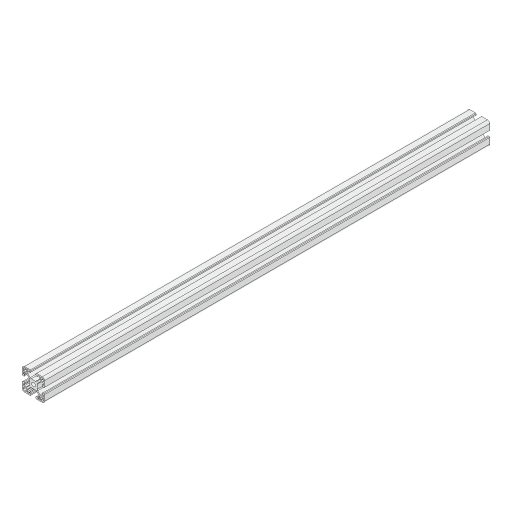
# Autodesk Inventor part: Al-profile-30x30
Saved by Autodesk Inventor 2023.1 (Build 271208000, 208)
## iProperties
Created: 2023-06-30
Part Number: Al-profile-30x30
Material: Aluminum 6061
Document SubType Name: Modeling
Designer: kuzmin
Density: 2.7 g/cm^3
Appearance: Aluminum - Flat
length: 600.000 mm
Author: kuzmin
Autodesk Inventor part; units mm, degrees
ref_plane "YZ Plane" through (0, 0, 0) normal (1, 0, 0) x (0, 1, 0)
ref_plane "XZ Plane" through (0, 0, 0) normal (0, 1, 0) x (-1, 0, 0)
ref_plane "XY Plane" through (0, 0, 0) normal (0, 0, 1) x (1, 0, 0)
sketch "Sketch1" plane through (0, 0, 0) normal (0, 0, 1) x (1, 0, 0)
  line L0 (5.2, -2.9574) -> (5.2, 2.9574) construction
  arc A0 (5.7858, 4.3716) -> (5.2, 2.9574) centre (7.2, 2.9574) ccw
  line L1 (5.7858, 4.3716) -> (9.0284, 7.6142)
  arc A1 (10.4426, 8.2) -> (9.0284, 7.6142) centre (10.4426, 6.2) ccw
  line L2 (10.4426, 8.2) -> (12.8, 8.2)
  arc A2 (13.6, 7.4) -> (12.8, 8.2) centre (12.8, 7.4) ccw
  line L3 (13.6, 7.4) -> (13.6, 6.1)
  arc A3 (13.3, 5.8) -> (13.6, 6.1) centre (13.3, 6.1) ccw
  line L4 (13.3, 5.8) -> (12.25, 5.8)
  arc A4 (12.25, 5.8) -> (11.95, 5.5) centre (12.25, 5.5) ccw
  line L5 (11.95, 5.5) -> (11.95, 4.2)
  arc A5 (11.95, 4.2) -> (12.75, 3.4) centre (12.75, 4.2) ccw
  line L6 (12.75, 3.4) -> (14.2, 3.4)
  arc A6 (14.2, 3.4) -> (15, 4.2) centre (14.2, 4.2) ccw
  line L7 (15, 4.2) -> (15, 12)
  arc A7 (15, 12) -> (12, 15) centre (12, 12) ccw
  line L8 (12, 15) -> (4.2, 15)
  arc A8 (4.2, 15) -> (3.4, 14.2) centre (4.2, 14.2) ccw
  line L9 (3.4, 14.2) -> (3.4, 12.75)
  arc A9 (3.4, 12.75) -> (4.2, 11.95) centre (4.2, 12.75) ccw
  line L10 (4.2, 11.95) -> (5.5, 11.95)
  arc A10 (5.5, 11.95) -> (5.8, 12.25) centre (5.5, 12.25) ccw
  line L11 (5.8, 12.25) -> (5.8, 13.3)
  arc A11 (6.1, 13.6) -> (5.8, 13.3) centre (6.1, 13.3) ccw
  line L12 (6.1, 13.6) -> (7.4, 13.6)
  arc A12 (8.2, 12.8) -> (7.4, 13.6) centre (7.4, 12.8) ccw
  line L13 (8.2, 12.8) -> (8.2, 10.4426)
  arc A13 (7.6142, 9.0284) -> (8.2, 10.4426) centre (6.2, 10.4426) ccw
  line L14 (7.6142, 9.0284) -> (4.3716, 5.7858)
  arc A14 (2.9574, 5.2) -> (4.3716, 5.7858) centre (2.9574, 7.2) ccw
  line L15 (2.9574, 5.2) -> (-2.9574, 5.2) construction
  circle A15 centre (0, 0) radius 2.575
  line L16 (12, 13.5) -> (9.9, 13.5)
  arc A16 (13.5, 12) -> (12, 13.5) centre (12, 12) ccw
  line L17 (13.5, 9.9) -> (13.5, 12)
  arc A17 (13.2, 9.6) -> (13.5, 9.9) centre (13.2, 9.9) ccw
  line L18 (9.9, 9.6) -> (13.2, 9.6)
  arc A18 (9.6, 9.9) -> (9.9, 9.6) centre (9.9, 9.9) ccw
  line L19 (9.6, 13.2) -> (9.6, 9.9)
  arc A19 (9.9, 13.5) -> (9.6, 13.2) centre (9.9, 13.2) ccw
  line L20 (0, 0) -> (12.0091, 12.0091) construction
  line L21 (2.9574, 5.2) -> (5.2, 5.2) construction
  line L22 (5.2, 5.2) -> (5.2, 2.9574) construction
  line L23 (2.9574, 7.2) -> (7.2, 2.9574) construction
  line L24 (9.0284, 7.6142) -> (8.3213, 8.3213) construction
  line L25 (8.3213, 8.3213) -> (7.6142, 9.0284) construction
  line L26 (6.2, 10.4426) -> (10.4426, 6.2) construction
  line L27 (2.9574, 5.2) -> (0, 5.2)
  line L28 (0, 2.575) -> (0, 5.2)
  line L29 (2.575, 0) -> (5.2, 0)
  line L30 (5.2, 0) -> (5.2, 2.9574)
  point P0 (11.55, 9.6)
  point P1 (8.3213, 8.3213)
  point P2 (5.2, 2.9574)
  dimension "d2" = 5.9147
  dimension "d3" = 4.5858
  dimension "d20" = 1.4
  dimension "d21" = 1.4
  dimension "d23" = 5.15
  dimension "d31" = 7.8
  dimension "d32" = 2.1
  dimension "d33" = 2
  dimension "d34" = 3
  dimension "d35" = 7.8
  dimension "d36" = 0.8
  dimension "d37" = 0.8
  dimension "d38" = 0.3
  dimension "d39" = 0.8
  dimension "d40" = 0.3
  dimension "d41" = 0.3
  dimension "d42" = 1.5
  dimension "d43" = 0.3
  dimension "d44" = 0.8
  dimension "d45" = 0.3
  dimension "d46" = 2
  dimension "d47" = 0.3
  dimension "d48" = 0.8
  dimension "d49" = 0.8
  dimension "d50" = 0.3
  dimension "d51" = 1.3
  dimension "d52" = 1.45
  dimension "d53" = 5.2
  dimension "d54" = 5.2
  dimension "d55" = 2
  dimension "d56" = 2.1
  dimension "d57" = 3.3
  dimension "d58" = 1.3
  dimension "d59" = 1.3
  dimension "d60" = 1.05
  dimension "d61" = 1.45
  dimension "d62" = 1.3
  dimension "d63" = 1.05
  dimension "d64" = 2.3574
  dimension "d65" = 2.3574
  constraints: 62 end point, 41 point on circle, 38 tangent, 20 centre point, 9 horizontal, 6 vertical, 5 equal length, 4 midpoint, 4 perpendicular, 4 point on line, 1 coincident, 1 collinear
  measures "d2" distance of L0.start L0.end
  measures "d3" distance of L14.start L14.end
  measures "d20" distance from line of L2 point (11.55, 9.6)
  measures "d21" distance between parallel lines of L13 L19
  measures "d23" diameter of A15
  measures "d31" distance of L8.start L8.end
  measures "d32" distance of L16.start L16.end
  measures "d33" radius of A14
  measures "d34" radius of A7
  measures "d35" distance of L7.start L7.end
  measures "d36" radius of A6
  measures "d37" radius of A5
  measures "d38" radius of A4
  measures "d39" radius of A2
  measures "d40" radius of A18
  measures "d41" radius of A17
  measures "d42" radius of A16
  measures "d43" radius of A19
  measures "d44" radius of A12
  measures "d45" radius of A11
  measures "d46" radius of A1
  measures "d47" radius of A3
  measures "d48" radius of A8
  measures "d49" radius of A9
  measures "d50" radius of A10
  measures "d51" distance of L10.start L10.end
  measures "d52" distance of L9.start L9.end
  measures "d53" distance from line of L0 L20.start
  measures "d54" distance from line of L15 L20.start
  measures "d55" radius of A0
  measures "d56" distance of L17.start L17.end
  measures "d57" distance of L18.start L18.end
  measures "d58" distance of L3.start L3.end
  measures "d59" distance of L12.start L12.end
  measures "d60" distance of L4.start L4.end
  measures "d61" distance of L6.start L6.end
  measures "d62" distance of L5.start L5.end
  measures "d63" distance of L11.start L11.end
  measures "d64" distance of L13.start L13.end
  measures "d65" distance of L2.start L2.end
extrude "Extrusion1" add sketch "Sketch1" along normal blind 600 contours A0 L30 L29 A15 L28 L27 A14 L14 A13 L13 A12 L12 A11 L11 A10 L10 A9 L9 A8 L8 A7 L7 A6 L6 A5 L5 A4 L4 A3 L3 A2 L2 A1 L1
pattern_circular "Circular Pattern1" count 4 over 360 about axis through (0, 0, -10) along (0, 0, 1) of "Extrusion1"
equation "\"length\" = 600"
body "Solid1"
